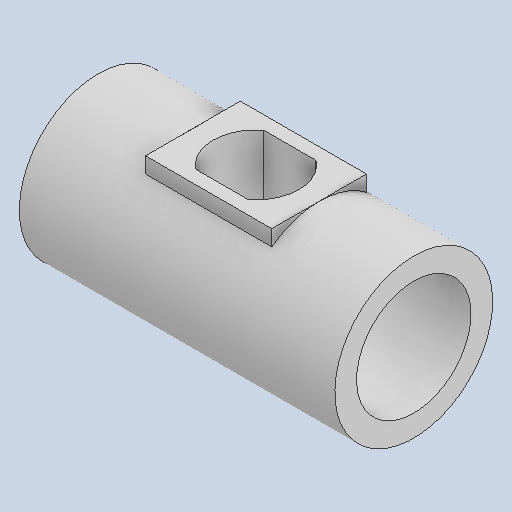
# Autodesk Inventor part: part_holder
Saved by Autodesk Inventor 2025 (Build 290162000, 162)
## iProperties
Created: 2025-07-16
Part Number: part_holder
Material: Generic
Document SubType Name: Modeling
Designer: Pravoslav
Density: 1 g/cm^3
Appearance: Default
Author: Pravoslav
Autodesk Inventor part; units mm, degrees
ref_plane "YZ Plane" through (0, 0, 0) normal (1, 0, 0) x (0, 1, 0)
ref_plane "XY Plane" through (0, 0, 0) normal (0, 0, 1) x (1, 0, 0)
sketch "Sketch1" plane through (0, 0, 0) normal (1, 0, 0) x (0, 1, 0)
  circle A0 centre (0, 0) radius 3.625
  circle A1 centre (0, 0) radius 5
  dimension "d0" = 7.25
  dimension "d1" = 10
  constraints: 2 centre point, 2 coincident
  measures "d0" diameter of A0
  measures "d1" diameter of A1
extrude "Extrusion1" add sketch "Sketch1" along normal mid plane 20
ref_plane "Work Plane1" through (0, 5, 0) normal (0, 1, 0) x (-1, 0, 0)
sketch "Sketch2" plane through (0, 5, 0) normal (0, 1, 0) x (-1, 0, 0)
  line L0 (-1.65, 2.15) -> (1.65, 2.15)
  line L1 (1.65, 2.15) -> (1.65, -2.15)
  line L2 (1.65, -2.15) -> (-1.65, -2.15)
  line L3 (-1.65, -2.15) -> (-1.65, 2.15)
  line L4 (-1.65, 2.15) -> (1.65, -2.15) construction
  line L5 (1.65, 2.15) -> (-1.65, -2.15) construction
  line L6 (-4, 3) -> (4, 3)
  line L7 (4, 3) -> (4, -3)
  line L8 (4, -3) -> (-4, -3)
  line L9 (-4, -3) -> (-4, 3)
  line L10 (-4, 3) -> (4, -3) construction
  line L11 (4, 3) -> (-4, -3) construction
  arc A0 (1.65, -2.15) -> (1.65, 2.15) centre (0.0168, 0) ccw
  arc A1 (-1.65, 2.15) -> (-1.65, -2.15) centre (-0.0168, 0) ccw
  point P0 (0, 0)
  dimension "d4" = 3.3
  dimension "d5" = 4.3
  dimension "d9" = 8
  dimension "d10" = 6
  dimension "d15" = 2.7
  dimension "d16" = 2.7
  constraints: 24 end point, 4 midpoint, 4 parallel, 4 point on circle, 2 centre point, 2 horizontal, 2 perpendicular
  measures "d4" distance of L1.end L2.end
  measures "d5" distance of L0.end L1.end
  measures "d9" distance of L7.end L8.end
  measures "d10" distance of L6.end L7.end
  measures "d15" radius of A0
  measures "d16" radius of A1
extrude "Extrusion2" add sketch "Sketch2" against normal blind 4.125 contours L0 L1 L2 L3 | L3 A1 | A0 L1 | L6 L7 L8 L9
extrude "Extrusion3" cut sketch "Sketch2" against normal up to surface (4.125 mm away) contours L0 L1 L2 L3 | L3 A1 | A0 L1
body "Solid1"
